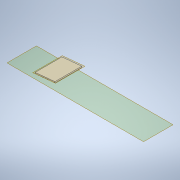
# Autodesk Inventor part: arc n°2
Saved by Autodesk Inventor 2020.2 (Build 242310000, 310)
## iProperties
Created: 2020-01-28
Part Number: arc n°2
Material: Générique
Document SubType Name: Modeling
Designer: anton
Density: 1 g/cm^3
Appearance: Par défaut
Author: anton
Autodesk Inventor part; units mm, degrees
ref_plane "YZ Plane" through (0, 0, 0) normal (1, 0, 0) x (0, 1, 0)
ref_plane "XZ Plane" through (0, 0, 0) normal (0, 1, 0) x (-1, 0, 0)
ref_plane "XY Plane" through (0, 0, 0) normal (0, 0, 1) x (1, 0, 0)
sketch "Esquisse1" plane through (0, 0, 0) normal (0, 0, 1) x (1, 0, 0)
  line L0 (-150.5839, 785.7) -> (150.5839, 785.7)
  arc A0 (150.5839, 785.7) -> (-150.5839, 785.7) centre (0, 0) ccw
  line L1 (-150.5839, 782.7) -> (150.5839, 782.7)
  arc A1 (150.5839, 782.7) -> (-150.5839, 782.7) centre (0, -3) ccw
  line L2 (-150.5839, 785.7) -> (-150.5839, 782.7)
  line L3 (150.5839, 785.7) -> (150.5839, 782.7)
  point P0 (0, 0)
  dimension "d4" = 785.7
  dimension "d8" = 3
  constraints: 8 end point, 4 point on circle, 2 centre point, 2 horizontal, 1 perpendicular
  measures "d4" distance from line of point (0, 0) L0
  measures "d8" distance between parallel lines of L0 L1
extrude "Extrusion1" add sketch "Esquisse1" along normal blind 65 contours A0 L0 A1 | L0 A1 L2 | L3 A1 L0
ref_plane "Plan de construction1" through (-150.5839, 782.7, 65) normal (0, -1, 0) x (0, 0, -1)
sketch "Esquisse2" plane through (-150.5839, 782.7, 65) normal (0, -1, 0) x (0, 0, -1)
  line L0 (65, 0) -> (0, 0) projected
  line L1 (0, 0) -> (65, 0)
  line L2 (65, 0) -> (65, 50)
  line L3 (65, 50) -> (0, 50)
  line L4 (0, 50) -> (0, 0)
  line L5 (0, 0) -> (0, 301.1678) projected
  line L6 (0, 301.1678) -> (65, 301.1678)
  line L7 (65, 301.1678) -> (65, 98)
  line L8 (65, 98) -> (0, 98)
  line L9 (0, 98) -> (0, 301.1678)
  line L10 (0, 50) -> (65, 50)
  line L11 (65, 50) -> (65, 98)
  line L12 (65, 98) -> (0, 98)
  line L13 (0, 98) -> (0, 50)
  point P0 (65, 150.5839)
  point P1 (0, 98)
  dimension "d13" = 50
  dimension "d14" = 48
  constraints: 24 end point, 6 parallel, 3 horizontal, 3 perpendicular, 1 point on line
  measures "d13" distance of L3.end L0.end
  measures "d14" distance between parallel lines of L8 L3
extrude "Extrusion2" cut sketch "Esquisse2" against normal through all contours L0 L4 L3 L2 | L8 L5 L6 L7
ref_plane "Plan de construction2" through (-100.5839, 793.6516, 65) normal (-0.0957734, 0.9954032, 0) x (0.9954032, 0.0957734, 0)
sketch "Esquisse3" plane through (-100.5839, 793.6516, 65) normal (-0.0957734, 0.9954032, 0) x (0.9954032, 0.0957734, 0)
  line L0 (47.9343, 65) -> (-0.2873, 65) projected
  line L1 (0, 0) -> (48.2217, 0) projected
  line L2 (-0.2873, 65) -> (48.2217, 65)
  line L3 (48.2217, 65) -> (48.2217, 0)
  line L4 (48.2217, 0) -> (-0.2873, 0)
  line L5 (-0.2873, 0) -> (-0.2873, 65)
  point P0 (24.1108, 65)
  point P1 (0, 0)
  constraints: 8 end point, 2 parallel, 1 horizontal, 1 perpendicular
extrude "Extrusion3" cut sketch "Esquisse3" along normal blind 10
